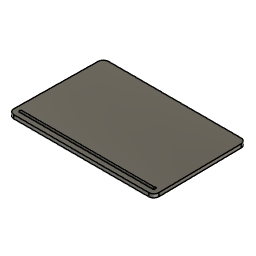
SeparatoreCassettaRossa v2 (Autodesk Fusion 360 design; units mm, degrees)
Autodesk Fusion 360 part; units mm, degrees
sketch "Schizzo1" plane through (0, 0, 0) normal (0, 0, 1) x (1, 0, 0)
  line L0 (-50, 0) -> (7.5, 0)
  line L1 (-49.5, 37) -> (-50, 0)
  line L2 (7, 37) -> (7.5, 0)
  line L3 (-49.5, 37) -> (7, 37)
  dimension "d7" = 57.5
  constraint horizontal L0
  measures "d7" distance of L0.start L0.end
extrude "Estrusione1" add sketch "Schizzo1" along normal blind 1.4
fillet "Raccordo1" radius 2 4 edges at (-50, 0, 0.7) (-49.5, 37, 0.7) (7, 37, 0.7) (7.5, 0, 0.7)
sketch "Schizzo2" plane through (0, 0, 1.4) normal (0, 0, 1) x (-1, 0, 0)
  line L0 (47.9728, 0) -> (-5.4728, 0)
  line L1 (-7.4726, -2.027) -> (-7.0267, -35.027)
  line L2 (-5.0268, -37) -> (47.5268, -37)
  line L3 (49.5267, -35.027) -> (49.9726, -2.027)
  arc A0 (-5.4728, 0) -> (-7.4726, -2.027) centre (-5.4728, -2) ccw
  arc A1 (-7.0267, -35.027) -> (-5.0268, -37) centre (-5.0268, -35) ccw
  arc A2 (47.5268, -37) -> (49.5267, -35.027) centre (47.5268, -35) ccw
  arc A3 (49.9726, -2.027) -> (47.9728, 0) centre (47.9728, -2) ccw
  line L4 (-5.4728, -2) -> (48, -2)
  line L5 (48, -2) -> (48, -3)
  line L6 (48, -3) -> (-5.4728, -3)
  line L7 (-5.4728, -3) -> (-5.4728, -2)
  constraint horizontal L4
  constraint vertical L5
  constraint horizontal L6
  constraint vertical L7
  constraint coincident A0.centre L4.start
extrude "Estrusione2" add sketch "Schizzo2" along normal blind 0.5 contours L4 L5 L6 L7
fillet "Raccordo2" radius 0.5 4 edges at (-21.2636, 3, 1.9) (-21.2636, 2, 1.9) (5.4728, 2.5, 1.9) (-48, 2.5, 1.9)
